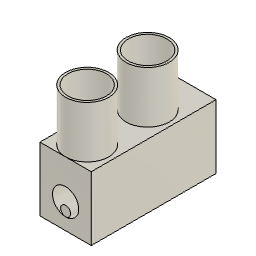
platinum_silver_electrode v9 (Autodesk Fusion 360 archive; units mm, degrees)
design "cable_terminal"
Autodesk Fusion 360 part; units mm, degrees
sketch "Sketch1" plane through (0, 0, 0) normal (0, 1, 0) x (1, 0, 0)
  circle A0 centre (0, 0) radius 0.65
  line L0 (0, 0) -> (0, -1.05) construction
  circle A1 centre (0, -1.05) radius 1.7
  line L1 (0, -1.05) -> (0, 2.22) construction
  line L2 (0, 2.22) -> (0, -1.93) construction
  line L3 (3.33, 2.22) -> (-3.33, 2.22)
  line L4 (-3.33, 2.22) -> (-3.33, -6.08)
  line L5 (-3.33, -6.08) -> (3.33, -6.08)
  line L6 (3.33, -6.08) -> (3.33, 2.22)
  line L7 (3.33, 2.22) -> (-3.33, -6.08) construction
  line L8 (-3.33, 2.22) -> (3.33, -6.08) construction
  point P0 (0, -1.93)
  dimension "d1" = 1.3
  dimension "d2" = 1.05
  dimension "d3" = 3.4
  dimension "d4" = 3.27
  dimension "d5" = 4.15
  dimension "d6" = 6.66
  dimension "d7" = 8.3
  constraint coincident A0.centre L0.start
  constraint vertical L0
  constraint coincident L0.end A1.centre
  constraint parallel L0 L1
  constraint parallel L1 L2
  constraint horizontal L3
  constraint perpendicular L3 L4
  constraint parallel L3 L5
  constraint parallel L4 L6
  constraint coincident L7 P0
  constraint coincident L8 P0
  constraint coincident P0 L2.end
  measures "d1" diameter of A0
  measures "d2" distance of A0.centre L0.end
  measures "d3" diameter of A1
  measures "d4" distance of L0.end L1.end
  measures "d5" distance of L1.end P0
  measures "d6" distance of L4.end L5.end
  measures "d7" distance of L3.end L4.end
extrude "Extrude1" add sketch "Sketch1" along normal blind 16.2
sketch "Sketch2" plane through (0, 0, 6.08) normal (0, 0, 1) x (-1, 0, 0)
  line L0 (3.33, 0) -> (-3.33, 0)
  line L1 (-3.33, 0) -> (-3.33, -16.2)
  line L2 (-3.33, -16.2) -> (3.33, -16.2)
  line L3 (3.33, -16.2) -> (3.33, 0)
  line L4 (0, 0) -> (0, -2.8) construction
  circle A0 centre (0, -2.8) radius 2.8
  circle A1 centre (0, -2.8) radius 2.5
  line L5 (0, -16.2) -> (0, -10.65) construction
  circle A2 centre (0, -10.65) radius 2.8
  circle A3 centre (0, -10.65) radius 2.5
  dimension "d10" = 2.8
  dimension "d11" = 5.6
  dimension "d12" = 5
  dimension "d13" = 5.55
  dimension "d14" = 5.6
  dimension "d15" = 5
  constraint coincident L4.start origin
  constraint perpendicular L0 L4
  constraint coincident L4.end A0.centre
  constraint concentric A0 A1
  constraint midpoint L2 L5.start
  constraint perpendicular L2 L5
  constraint coincident L5.end A2.centre
  constraint concentric A2 A3
  measures "d10" distance of L4.start L4.end
  measures "d11" diameter of A0
  measures "d12" diameter of A1
  measures "d13" distance of L5.start L5.end
  measures "d14" diameter of A2
  measures "d15" diameter of A3
extrude "Extrude2" add sketch "Sketch2" along normal blind 6.7 contours A0 | A2
equation "d2 = ( 3.4 / 2 ) * 1 mm - ( 1.3 / 2 ) * 1 mm"
equation "d4 = ( 3.4 / 2 ) * 1 mm + 1.57 mm"
equation "d5 = ( 8.3 / 2 ) * 1 mm"
equation "d16 = 15 mm - 8.3 mm"

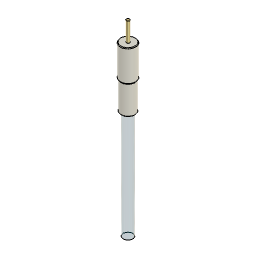
design "silver_reference_electrode"
Autodesk Fusion 360 part; units mm, degrees
sketch "Sketch1" plane through (0, 0, 0) normal (0, 0, 1) x (1, 0, 0)
  circle A0 centre (0, 0) radius 0.65
  dimension "d1" = 1.3
  constraint coincident A0.centre origin
  measures "d1" diameter of A0
extrude "Extrude1" add sketch "Sketch1" against normal blind 8 makes body 1
sketch "Sketch2" plane through (0, 0, -8) normal (0, 0, -1) x (1, 0, 0)
  circle A0 centre (0, 0) radius 0.65
  circle A1 centre (0, 0) radius 3.175
  dimension "d4" = 6.35
  constraint coincident A0.centre A1.centre
  measures "d4" diameter of A1
extrude "Extrude2" add sketch "Sketch2" along normal blind 13 separate body contours A0 | A1 makes body 2
sketch "Sketch3" plane through (0, 0, -21) normal (0, 0, -1) x (1, 0, 0)
  circle A0 centre (0, 0) radius 3.175
  circle A1 centre (0, 0) radius 2.9
  dimension "d7" = 5.8
  constraint coincident A0.centre A1.centre
  measures "d7" diameter of A1
extrude "Extrude3" add sketch "Sketch3" along normal blind 12 contours A1 bodies 2
sketch "Sketch4" plane through (0, 0, -33) normal (0, 0, -1) x (1, 0, 0)
  circle A0 centre (0, 0) radius 2.9
  circle A1 centre (0, 0) radius 2
  dimension "d10" = 4
  constraint coincident A0.centre A1.centre
  measures "d10" diameter of A1
extrude "Extrude4" add sketch "Sketch4" along normal blind 45 separate body contours A1 makes body 3
fillet "Fillet1" radius 0.25 1 edges at (-2.9601, 1.1481, -21) on bodies 2
fillet "Fillet2" radius 0.25 1 edges at (-2.7037, -1.0487, -21) on bodies 2
fillet "Fillet3" radius 0.25 1 edges at (-2.7037, 1.0487, -33) on bodies 2
fillet "Fillet4" radius 0.25 1 edges at (-2.9601, 1.1481, -8) on bodies 2
named bodies: "gold", "ptfe", "glass"
